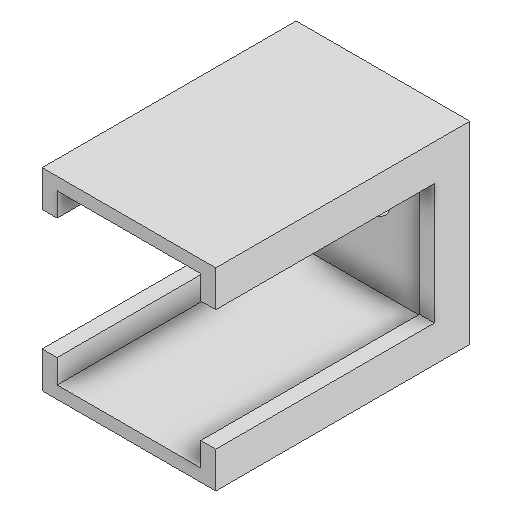
# Autodesk Inventor part: ARM_1 SKETCH
Saved by Autodesk Inventor 2025.3 (Build 293356030, 356C)
## iProperties
Created: 2025-09-30
Part Number: ARM_1 SKETCH
Material: 일반
Document SubType Name: Modeling
Designer: joseph
Density: 1 g/cm^3
Appearance: 기본값
Author: joseph
Autodesk Inventor part; units mm, degrees
ref_plane "XZ Plane" through (0, 0, 0) normal (0, 1, 0) x (-1, 0, 0)
ref_plane "XY Plane" through (0, 0, 0) normal (0, 0, 1) x (1, 0, 0)
ref_plane "작업 평면10" through (-23.2, 0, 152.9) normal (0, 0, 1) x (1, 0, 0)
sketch "스케치8" plane through (-23.2, 0, 152.9) normal (0, 0, 1) x (1, 0, 0)
  line L0 (17.25, -20.2) -> (-17.25, -20.2)
  line L1 (-17.25, -20.2) -> (-17.25, 20.2)
  line L2 (-17.25, 20.2) -> (17.25, 20.2)
  line L3 (17.25, 20.2) -> (17.25, -20.2)
  circle A0 centre (0, 0) radius 2 projected
  line L4 (-17.25, -20.2) -> (-12.65, -20.2)
  line L5 (-12.65, 20.2) -> (-17.25, 20.2)
  line L6 (-17.25, 20.2) -> (-17.25, -20.2)
  line L7 (17.25, -20.2) -> (12.65, -20.2)
  line L8 (12.65, -20.2) -> (12.65, 20.2)
  line L9 (12.65, 20.2) -> (17.25, 20.2)
  line L10 (17.25, 20.2) -> (17.25, -20.2)
  line L11 (17.25, 20.2) -> (20.85, 20.2)
  line L12 (20.85, 20.2) -> (20.85, -20.2)
  line L13 (20.85, -20.2) -> (17.25, -20.2)
  line L14 (17.25, -20.2) -> (17.25, 20.2)
  line L15 (-17.25, 20.2) -> (-12.65, 20.2)
  line L16 (-12.65, 20.2) -> (-12.65, -20.2)
  line L17 (-12.65, -20.2) -> (-17.25, -20.2)
  line L18 (-17.25, -20.2) -> (-17.25, 20.2)
  line L19 (-17.25, 20.2) -> (-20.85, 20.2)
  line L20 (-20.85, 20.2) -> (-20.85, -20.2)
  line L21 (-17.25, -20.2) -> (-17.25, 20.2)
  line L22 (20.85, 14.5) -> (17.25, 14.5)
  line L23 (17.25, 14.5) -> (17.25, -14.5)
  line L24 (17.25, -14.5) -> (20.85, -14.5)
  line L25 (20.85, -14.5) -> (20.85, 14.5)
  line L26 (0, -20.2) -> (0, 20.2) construction
  line L27 (-17.25, 20.2) -> (-17.25, -20.2)
  circle A1 centre (0, 0) radius 2
  line L28 (-17.25, -20.2) -> (-12.65, -20.2)
  line L29 (-12.65, -20.2) -> (-12.65, 20.2)
  line L30 (-12.65, 20.2) -> (-17.25, 20.2)
  line L31 (-17.25, 20.2) -> (-17.25, -20.2)
  line L32 (-17.25, 20.2) -> (-20.85, 20.2)
  line L33 (-20.85, 20.2) -> (-20.85, -20.2)
  line L34 (-17.25, -20.2) -> (-17.25, 20.2)
  line L35 (-20.85, 14.5) -> (-17.25, 14.5)
  line L36 (-17.25, 14.5) -> (-17.25, -14.5)
  line L37 (-17.25, -14.5) -> (-20.85, -14.5)
  line L38 (-20.85, -14.5) -> (-20.85, 14.5)
  line L39 (-20.85, 20.2) -> (20.85, 20.2)
  line L40 (20.85, 20.2) -> (20.85, 23.2)
  line L41 (20.85, 23.2) -> (-20.85, 23.2)
  line L42 (-20.85, 23.2) -> (-20.85, 20.2)
  line L43 (-17.25, -20.2) -> (-20.85, -20.2)
  line L44 (-20.85, -20.2) -> (20.85, -20.2)
  line L45 (20.85, -20.2) -> (20.85, -23.2)
  line L46 (20.85, -23.2) -> (-20.85, -23.2)
  line L47 (-20.85, -23.2) -> (-20.85, -20.2)
  point P0 (23.2, 0)
  point P1 (-17.25, 0)
  point P2 (20.85, 0)
  point P3 (-23.2, 0)
  point P4 (-20.85, 0)
  point P5 (17.25, 14.5)
  point P6 (20.85, -14.5)
  point P7 (17.25, -14.5)
  point P8 (-17.25, -14.5)
  point P9 (-20.85, -14.5)
  point P10 (-20.85, 14.5)
  point P11 (-17.25, 14.5)
  point P12 (-17.25, 20.2)
  point P13 (20.85, 20.2)
  point P14 (-17.25, 14.5)
  point P15 (-17.25, -14.5)
  point P16 (-20.85, -14.5)
  dimension "d27" = 34.5
  dimension "d30" = 4.6
  dimension "d33" = 29
  dimension "d34" = 40.4
  dimension "d48" = 3
  dimension "d53" = 3
  constraints: 96 end point, 16 parallel, 10 horizontal, 10 symmetric about line, 8 perpendicular, 6 point on line, 4 midpoint, 2 horizontal alignment, 1 centre point, 1 vertical, 1 vertical alignment, 1 other
  measures "d27" distance of L1.end L2.end
  measures "d30" distance of L8.end L9.end
  measures "d33" distance of L23.end L22.end
  measures "d34" distance of L11.end L12.end
  measures "d48" distance of L40.end L39.end
  measures "d53" distance of L44.end L45.end
extrude "돌출7" add sketch "스케치8" along normal blind 3 contours L0 L8 L2 L3 | L3 L24 L12 L13 | L0 L16 L2 L8 | L3 L22 L12 L24 | L0 L1 L2 L16 | L3 L11 L12 L22 | L43 L20 L37 L1 | L37 L20 L35 L1 | L1 L35 L20 L19
extrude "돌출8" add sketch "스케치8" along normal blind 61 contours L13 L45 L46 L47 L43 L0 | L3 L24 L12 L13 | L2 L19 L42 L41 L40 L11 | L3 L11 L12 L22 | L43 L20 L37 L1 | L1 L35 L20 L19
ref_plane "작업 평면3" through (-23.2, 0, 0) normal (1, 0, 0) x (0, 1, 0)
sketch "스케치10" plane through (-23.2, 0, 155.9) normal (0, 0, 1) x (1, 0, 0)
  line L0 (-17.25, -14.5) -> (-17.25, -20.2) projected
  line L1 (-17.25, -20.2) -> (17.25, -20.2) projected
  line L2 (17.25, -20.2) -> (17.25, -14.5) projected
  line L3 (17.25, -14.5) -> (20.85, -14.5) projected
  line L4 (20.85, -14.5) -> (20.85, 14.5) projected
  line L5 (20.85, 14.5) -> (17.25, 14.5) projected
  line L6 (17.25, 14.5) -> (17.25, 20.2) projected
  line L7 (17.25, 20.2) -> (-17.25, 20.2) projected
  circle A0 centre (0, 0) radius 2 projected
  line L8 (-20.85, -14.75) -> (-17.25, -14.75)
  line L9 (-17.25, -14.75) -> (-17.25, 14.75)
  line L10 (-17.25, 14.75) -> (-20.85, 14.75)
  line L11 (-20.85, 14.75) -> (-20.85, -14.75)
  line L12 (20.85, -14.5) -> (17.25, -14.5)
  line L13 (17.25, -14.5) -> (17.25, 14.5)
  line L14 (17.25, 14.5) -> (20.85, 14.5)
  line L15 (20.85, 14.5) -> (20.85, -14.5)
  line L16 (-17.25, 20.2) -> (-17.25, 14.5) projected
  line L17 (-17.25, 14.5) -> (-20.85, 14.5) projected
  line L18 (-20.85, 14.5) -> (-20.85, -14.5) projected
  line L19 (-20.85, -14.5) -> (-17.25, -14.5) projected
  point P0 (23.2, 0)
  constraints: 16 end point, 4 parallel, 2 horizontal, 2 perpendicular
extrude "돌출10" add sketch "스케치10" along normal blind 5.5 contours L19 L11 L17 L9 | L0 L8 L11 L19 | L17 L11 L10 L9 | L13 L5 L4 L3
sketch "스케치11" plane through (-23.2, 0, 155.9) normal (0, 0, 1) x (1, 0, 0)
  circle A0 centre (0, 0) radius 5
  point P0 (23.2, 0)
  dimension "d54" = 10
  constraints: 1 centre point
  measures "d54" diameter of A0
extrude "돌출11" cut sketch "스케치11" against normal blind 5.5
